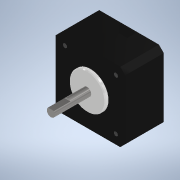
# Autodesk Inventor part: KTC-5017-010
Saved by Autodesk Inventor 2020 (Build 240168000, 168)
## iProperties
Created: 2014-01-06
Part Number: KTC-5017-010
Material: Steel, Carbon
Document SubType Name: Modeling
Designer: Vinicius
Density: 7.87 g/cm^3
Appearance: Smooth - Black
Mass: 552.982 g
Surface Area: 115.114 cm^2
Volume: 70.2645 cm^3
Author: Vinicius
Title: Motor de passo nema 17 - 3.1 Kgf/cm KCT-5017-010
Autodesk Inventor part; units mm, degrees
ref_plane "YZ Plane" through (0, 0, 0) normal (1, 0, 0) x (0, 1, 0)
ref_plane "XZ Plane" through (0, 0, 0) normal (0, 1, 0) x (-1, 0, 0)
ref_plane "XY Plane" through (0, 0, 0) normal (0, 0, 1) x (1, 0, 0)
sketch "Sketch1" plane through (0, 0, 0) normal (0, 0, 1) x (1, 0, 0)
  line L0 (-18.15, 21.15) -> (18.15, 21.15)
  line L1 (21.15, 18.15) -> (21.15, -18.15)
  line L2 (18.15, -21.15) -> (-18.15, -21.15)
  line L3 (-21.15, -18.15) -> (-21.15, 18.15)
  line L4 (-21.15, 21.15) -> (21.15, -21.15) construction
  line L5 (21.15, 21.15) -> (-21.15, -21.15) construction
  line L6 (18.15, 21.15) -> (21.15, 18.15)
  line L7 (-18.15, 21.15) -> (-21.15, 18.15)
  line L8 (-21.15, -18.15) -> (-18.15, -21.15)
  line L9 (18.15, -21.15) -> (21.15, -18.15)
  line L10 (-15.5, 15.5) -> (15.5, 15.5) construction
  line L11 (15.5, 15.5) -> (15.5, -15.5) construction
  line L12 (15.5, -15.5) -> (-15.5, -15.5) construction
  line L13 (-15.5, -15.5) -> (-15.5, 15.5) construction
  line L14 (-15.5, 15.5) -> (15.5, -15.5) construction
  line L15 (15.5, 15.5) -> (-15.5, -15.5) construction
  circle A0 centre (-15.5, 15.5) radius 1.5
  circle A1 centre (15.5, 15.5) radius 1.5
  circle A2 centre (15.5, -15.5) radius 1.5
  circle A3 centre (-15.5, -15.5) radius 1.5
  point P0 (0, 0)
  dimension "d0" = 42.3
  dimension "d1" = 42.3
  dimension "d2" = 3
  dimension "d3" = 3
  dimension "d4" = 3
  dimension "d5" = 3
  dimension "d6" = 3
  dimension "d7" = 3
  dimension "d8" = 3
  dimension "d9" = 3
  dimension "d10" = 31
  dimension "d11" = 31
  dimension "d12" = 3
  dimension "d13" = 3
  dimension "d14" = 3
  dimension "d15" = 3
  constraints: 32 end point, 8 point on line, 4 centre point, 4 coincident, 4 midpoint, 4 parallel, 2 horizontal, 2 perpendicular
  measures "d0" distance of L4.end L5.end
  measures "d1" distance of L5.start L4.end
  measures "d2" distance of L0.end L5.start
  measures "d3" distance of L1.start L5.start
  measures "d4" distance of L0.start L4.start
  measures "d5" distance of L3.end L4.start
  measures "d6" distance of L3.start L5.end
  measures "d7" distance of L2.end L5.end
  measures "d8" distance of L2.start L4.end
  measures "d9" distance of L1.end L4.end
  measures "d10" distance of L11.end L12.end
  measures "d11" distance of L10.end L11.end
  measures "d12" diameter of A0
  measures "d13" diameter of A1
  measures "d14" diameter of A2
  measures "d15" diameter of A3
extrude "Extrusion1" add sketch "Sketch1" along normal blind 10
sketch "Sketch2" plane through (0, 0, 10) normal (0, 0, 1) x (1, 0, 0)
  line L0 (-18.15, 21.15) -> (18.15, 21.15)
  line L1 (21.15, 18.15) -> (21.15, -18.15)
  line L2 (18.15, -21.15) -> (-18.15, -21.15)
  line L3 (-21.15, -18.15) -> (-21.15, 18.15)
  line L4 (-21.15, 21.15) -> (21.15, -21.15) construction
  line L5 (21.15, 21.15) -> (-21.15, -21.15) construction
  line L6 (-18.15, 21.15) -> (-21.15, 18.15)
  line L7 (-21.15, -18.15) -> (-18.15, -21.15)
  line L8 (21.15, -18.15) -> (18.15, -21.15)
  line L9 (18.15, 21.15) -> (21.15, 18.15)
  point P0 (0, 0)
  dimension "d18" = 42.3
  dimension "d19" = 42.3
  dimension "d20" = 3
  dimension "d21" = 3
  dimension "d22" = 3
  dimension "d23" = 3
  dimension "d24" = 3
  dimension "d25" = 3
  dimension "d26" = 3
  dimension "d27" = 3
  constraints: 20 end point, 8 point on line, 2 midpoint, 2 parallel, 1 horizontal, 1 perpendicular
  measures "d18" distance of L4.end L5.end
  measures "d19" distance of L5.start L4.end
  measures "d20" distance of L0.start L4.start
  measures "d21" distance of L3.end L4.start
  measures "d22" distance of L3.start L5.end
  measures "d23" distance of L2.end L5.end
  measures "d24" distance of L1.end L4.end
  measures "d25" distance of L2.start L4.end
  measures "d26" distance of L0.end L5.start
  measures "d27" distance of L1.start L5.start
extrude "Extrusion2" add sketch "Sketch2" along normal blind 3.5
sketch "Sketch3" plane through (0, 0, 13.5) normal (0, 0, 1) x (1, 0, 0)
  line L0 (-18.15, 21.15) -> (18.15, 21.15)
  line L1 (21.15, 18.15) -> (21.15, -18.15)
  line L2 (18.15, -21.15) -> (-18.15, -21.15)
  line L3 (-21.15, -18.15) -> (-21.15, 18.15)
  line L4 (-21.15, 21.15) -> (21.15, -21.15) construction
  line L5 (21.15, 21.15) -> (-21.15, -21.15) construction
  line L6 (-18.15, 21.15) -> (-21.15, 18.15)
  line L7 (-21.15, -18.15) -> (-18.15, -21.15)
  line L8 (21.15, -18.15) -> (18.15, -21.15)
  line L9 (18.15, 21.15) -> (21.15, 18.15)
  line L10 (-15.5, 15.5) -> (15.5, 15.5) construction
  line L11 (15.5, 15.5) -> (15.5, -15.5) construction
  line L12 (15.5, -15.5) -> (-15.5, -15.5) construction
  line L13 (-15.5, -15.5) -> (-15.5, 15.5) construction
  line L14 (-15.5, 15.5) -> (15.5, -15.5) construction
  line L15 (15.5, 15.5) -> (-15.5, -15.5) construction
  circle A0 centre (-15.5, 15.5) radius 0.5
  circle A1 centre (-15.5, -15.5) radius 0.5
  circle A2 centre (15.5, -15.5) radius 0.5
  circle A3 centre (15.5, 15.5) radius 0.5
  point P0 (0, 0)
  dimension "d30" = 42.3
  dimension "d31" = 42.3
  dimension "d32" = 3
  dimension "d33" = 3
  dimension "d34" = 3
  dimension "d35" = 3
  dimension "d36" = 3
  dimension "d37" = 3
  dimension "d38" = 3
  dimension "d39" = 3
  dimension "d40" = 31
  dimension "d41" = 31
  dimension "d42" = 1
  dimension "d43" = 1
  dimension "d44" = 1
  dimension "d45" = 1
  constraints: 32 end point, 8 point on line, 4 centre point, 4 coincident, 4 midpoint, 4 parallel, 2 horizontal, 2 perpendicular
  measures "d30" distance of L4.end L5.end
  measures "d31" distance of L5.start L4.end
  measures "d32" distance of L0.start L4.start
  measures "d33" distance of L3.end L4.start
  measures "d34" distance of L3.start L5.end
  measures "d35" distance of L2.end L5.end
  measures "d36" distance of L1.end L4.end
  measures "d37" distance of L2.start L4.end
  measures "d38" distance of L0.end L5.start
  measures "d39" distance of L1.start L5.start
  measures "d40" distance of L11.end L12.end
  measures "d41" distance of L10.end L11.end
  measures "d42" diameter of A0
  measures "d43" diameter of A1
  measures "d44" diameter of A2
  measures "d45" diameter of A3
extrude "Extrusion3" add sketch "Sketch3" along normal blind 10
sketch "Sketch4" plane through (0, 0, 23.5) normal (0, 0, 1) x (1, 0, 0)
  circle A0 centre (0, 0) radius 11
  dimension "d48" = 22
  constraints: 1 centre point, 1 coincident
  measures "d48" diameter of A0
extrude "Extrusion4" add sketch "Sketch4" along normal blind 2
chamfer "Chamfer1" distance 0.5 angle 45 1 edges at (-11, 0, 25.5)
sketch "Sketch5" plane through (0, 0, 25.5) normal (0, 0, 1) x (1, 0, 0)
  circle A0 centre (0, 0) radius 10.5 projected
  circle A1 centre (0, 0) radius 2.5
  dimension "d54" = 5
  constraints: 1 centre point, 1 coincident
  measures "d54" diameter of A1
extrude "Extrusion5" add sketch "Sketch5" along normal blind 22 contours A1
sketch "Sketch6" plane through (-18.15, 21.15, 0) normal (0, 1, 0) x (1, 0, 0)
  line L0 (0, 0) -> (36.3, 0) projected
  line L1 (13.15, -1) -> (23.15, -1)
  line L2 (23.15, -1) -> (23.15, -9)
  line L3 (23.15, -9) -> (13.15, -9)
  line L4 (13.15, -9) -> (13.15, -1)
  line L5 (13.15, -1) -> (23.15, -9) construction
  line L6 (23.15, -1) -> (13.15, -9) construction
  point P0 (18.15, 0)
  point P1 (18.15, -5)
  dimension "d57" = 10
  dimension "d58" = 8
  dimension "d59" = 0
  dimension "d60" = 5
  constraints: 12 end point, 2 midpoint, 2 parallel, 1 horizontal, 1 perpendicular
  measures "d57" distance of L2.end L3.end
  measures "d58" distance of L1.end L2.end
  measures "d59" horizontal distance of point (18.15, 0) point (18.15, -5)
  measures "d60" distance from line of L0 point (18.15, -5)
extrude "Extrusion6" cut sketch "Sketch6" against normal blind 5
sketch "Sketch7" plane through (0, 0, 47.5) normal (0, 0, 1) x (1, 0, 0)
  circle A0 centre (0, 0) radius 2.5 projected
  arc A1 (1.8231, 1.7107) -> (-1.8197, 1.7142) centre (0, 0) ccw
  line L0 (-1.8197, 1.7142) -> (1.8231, 1.7107)
  dimension "d63" = 3.6428
  constraints: 4 point on circle, 2 end point, 1 centre point, 1 coincident, 1 concentric
  measures "d63" distance of L0.start L0.end
extrude "Extrusion7" cut sketch "Sketch7" against normal blind 10 contours L0 A0 picked at (0.4606, 1.8369)
sketch "Esboço10" plane through (0, 0, 23.5) normal (0, 0, 1) x (1, 0, 0)
  circle A0 centre (15.5, 15.5) radius 0.5 projected
  circle A1 centre (15.5, -15.5) radius 0.5 projected
  circle A2 centre (-15.5, -15.5) radius 0.5 projected
  circle A3 centre (-15.5, 15.5) radius 0.5 projected
  constraints: 4 coincident
hole "Furo1" at (-15.5, 15.5, 23.5) at (15.5, 15.5, 23.5) at (15.5, -15.5, 23.5) at (-15.5, -15.5, 23.5) direction (0, 0, -1) diameter 2.459 depth 6 tip angle 118 thread size "M3x0.5" class "6H" standard "ANSI Metric M Profile"
sketch "Sketch9" plane through (0, 0, 0) normal (0, 0, -1) x (-1, 0, 0)
  circle A0 centre (0, 0) radius 2.5
  dimension "d68" = 5
  constraints: 1 centre point, 1 coincident
  measures "d68" diameter of A0
equation "\"d3\" = d2"
equation "\"d4\" = d2"
equation "\"d5\" = d4"
equation "\"d6\" = d2"
equation "\"d7\" = d6"
equation "\"d8\" = d2"
equation "\"d9\" = d8"
equation "\"d21\" = d20"
equation "\"d23\" = d22"
equation "\"d24\" = d22"
equation "\"d25\" = d24"
equation "\"d26\" = d22"
equation "\"d27\" = d26"
equation "\"d33\" = d32"
equation "\"d34\" = d32"
equation "\"d35\" = d34"
equation "\"d36\" = d32"
equation "\"d37\" = d36"
equation "\"d38\" = d32"
equation "\"d39\" = d38"
body "Solid1"
